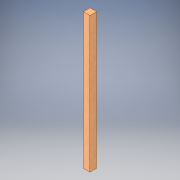
# Autodesk Inventor part: testsideLong
Saved by Autodesk Inventor 2019 (Build 230136000, 136)
## iProperties
Created: 2019-02-01
Part Number: testsideLong
Material: Wood (Cherry)
Document SubType Name: Modeling
Designer: gaincarlo
Density: 0.63 g/cm^3
Appearance: Cherry - Natural Low Gloss
Author: gaincarlo
Autodesk Inventor part; units mm, degrees
ref_plane "YZ Plane" through (0, 0, 0) normal (1, 0, 0) x (0, 1, 0)
ref_plane "XZ Plane" through (0, 0, 0) normal (0, 1, 0) x (-1, 0, 0)
ref_plane "XY Plane" through (0, 0, 0) normal (0, 0, 1) x (1, 0, 0)
sketch "Sketch1" plane through (0, 0, 0) normal (0, 1, 0) x (-1, 0, 0)
  line L0 (3, 3) -> (-17, 3)
  line L1 (-17, 3) -> (-17, -17)
  line L2 (-17, -17) -> (3, -17)
  line L3 (3, -17) -> (3, 3)
  point P0 (0, 0)
  dimension "d0" = 20
  dimension "d1" = 20
  constraints: 8 end point, 2 parallel, 1 horizontal, 1 perpendicular
  measures "d0" distance of L2.end L1.end
  measures "d1" distance of L1.end L0.end
extrude "Extrusion1" add sketch "Sketch1" along normal blind 410
body "Solid1"
